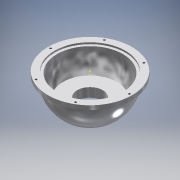
# Autodesk Inventor part: Kugel_unten_V5_leer
Saved by Autodesk Inventor 2016 (Build 200138000, 138)
## iProperties
Created: 2015-06-19
Part Number: Kugel_unten_V5_leer
Material: ABS-Kunststoff
Document SubType Name: Modeling
Designer: Johann
Mass: 41.0322 g
Surface Area: 192.915 cm^2
Volume: 38.7096 cm^3
Density: 1.06 g/cm^3
Appearance: Glatt - weiß
Author: Johann
Autodesk Inventor part; units mm, degrees
ref_plane "YZ Plane" through (0, 0, 0) normal (1, 0, 0) x (0, 1, 0)
sketch "Skizze1" plane through (0, 0, 0) normal (1, 0, 0) x (0, 1, 0)
  line L0 (0, 0) -> (0, 50)
  arc A0 (32.8487, 27.1754) -> (40, 50) centre (0, 50) ccw
  arc A1 (28.5, 15.1754) -> (45, 50) centre (0, 50) ccw
  line L1 (40, 50) -> (40, 55)
  line L2 (40, 55) -> (45, 55)
  line L3 (45, 55) -> (45, 50)
  line L4 (0, 50) -> (40, 50) construction
  line L5 (0, 50) -> (32.8487, 27.1754) construction
  line L6 (28.5, 15.1754) -> (22.5, 15.1754)
  line L7 (22.5, 15.1754) -> (22.5, 17.1754)
  line L8 (22.5, 17.1754) -> (18.5, 17.1754)
  line L9 (18.5, 17.1754) -> (18.5, 15.9754)
  line L10 (18.5, 15.9754) -> (15.5, 15.9754)
  line L11 (15.5, 15.9754) -> (15.5, 27.1754)
  line L12 (15.5, 27.1754) -> (32.8487, 27.1754)
  line L13 (0, 36.0806) -> (37.5, 36.0806) construction
  dimension "d3" = 5
  dimension "r_Kugel" = 45
  dimension "d5" = 50
  dimension "d7" = 5
  dimension "d36" = 4
  dimension "d38" = 2
  dimension "d40" = 1.2
  dimension "d41" = 45
  dimension "d179" = 3
  dimension "d194" = 17.3487
  dimension "d292" = 10
  dimension "d293" = 6
  dimension "d294" = 37.5
  dimension "d295" = 13.9194
  dimension "d296" = 8.9052
  constraints: 28 end point, 6 perpendicular, 6 point on circle, 4 horizontal, 3 coincident, 3 vertical, 2 centre point, 1 point on line, 1 tangent
  measures "d3" radial gap between concentric circles of A1 A0
  measures "r_Kugel" radius of A1
  measures "d5" distance of L0.start L0.end
  measures "d7" distance of L1.start L1.end
  measures "d36" distance of L7.end L8.end
  measures "d38" distance of L6.end L7.end
  measures "d40" distance of L8.end L9.end
  measures "d41" diameter of L7 L0
  measures "d179" distance of L9.end L10.end
  measures "d194" distance of L11.end L5.end
  measures "d292" distance between parallel lines of L12 L8
  measures "d293" distance of L6.start L6.end
  measures "d294" distance of L13.start L13.end
  measures "d295" distance between parallel lines of L4 L13
  measures "d296" distance between parallel lines of L12 L13
revolve "Umdrehung1" add sketch "Skizze1" angle 360 about axis through (0, 0, 0) along (0, 0, 1)
sketch "Skizze6" plane through (0, 0, 27.1754) normal (0, 0, 1) x (1, 0, 0)
  circle A0 centre (0, 0) radius 32.8487 construction
  circle A1 centre (0, 0) radius 15.5 construction
  line L0 (-6.5, -15.5) -> (18.5, -15.5)
  line L1 (18.5, -15.5) -> (18.5, -23.5)
  line L2 (18.5, -23.5) -> (-6.5, -23.5)
  line L3 (-6.5, -23.5) -> (-6.5, -15.5)
  line L4 (-6.5, -23.5) -> (18.5, -15.5) construction
  line L5 (18.5, -23.5) -> (-6.5, -15.5) construction
  circle A2 centre (0, 0) radius 32.8487 projected
  point P0 (0, 0)
  point P1 (6, -15.5)
  point P2 (6, -19.5)
  dimension "d130" = 8
  dimension "d180" = 25
  dimension "d191" = 6
  constraints: 12 end point, 2 midpoint, 2 parallel, 1 horizontal, 1 perpendicular, 1 tangent
  measures "d130" distance of L2.end L0.start
  measures "d180" distance of L0.start L0.end
  measures "d191" horizontal distance of point (0, 0) point (6, -19.5)
ref_plane "Arbeitsebene2" through (0, 0, 31.1754) normal (0, 0, 1) x (1, 0, 0)
sketch "Skizze7" plane through (0, 0, 31.1754) normal (0, 0, 1) x (1, 0, 0)
  line L0 (-6.5, -23.5) -> (-6.5, -15.5) construction
  line L1 (18.5, -23.5) -> (-6.5, -23.5) construction
  line L2 (-6.5, -15.5) -> (18.5, -15.5) construction
  line L3 (18.5, -15.5) -> (18.5, -23.5) construction
  line L4 (18.5, -23.5) -> (-6.5, -15.5) construction
  line L5 (-6.5, -23.5) -> (18.5, -15.5) construction
  line L6 (-0.5, -15.5) -> (19.5, -15.5)
  line L7 (19.5, -15.5) -> (19.5, -20.5)
  line L8 (19.5, -20.5) -> (-0.5, -20.5)
  line L9 (-0.5, -20.5) -> (-0.5, -15.5)
  line L10 (-0.5, -20.5) -> (19.5, -15.5) construction
  line L11 (19.5, -20.5) -> (-0.5, -15.5) construction
  point P0 (0, 0)
  point P1 (6, -19.5)
  point P2 (9.5, -15.5)
  point P3 (9.5, -18)
  dimension "d50" = 20
  dimension "d51" = 5
  dimension "d98" = 25
  dimension "d99" = 8
  dimension "d221" = 1
  constraints: 12 end point, 2 midpoint, 2 parallel, 1 collinear, 1 horizontal, 1 perpendicular
  measures "d50" distance of L7.end L8.end
  measures "d51" distance of L6.end L7.end
  measures "d98" distance of L1.start L0.start
  measures "d99" distance of L2.end L1.start
  measures "d221" distance between parallel lines of L7 L3
ref_plane "Arbeitsebene3" through (0, 0, 41.1754) normal (0, 0, 1) x (1, 0, 0)
sketch "Skizze8" plane through (0, 0, 41.1754) normal (0, 0, 1) x (1, 0, 0)
  point P0 (0, 0)
feature "Erhebung1" [suppressed]
extrude "Extrusion16" [suppressed]
feature "Rippe1" [suppressed]
sketch "Skizze31" plane through (-0.5, -20.5, 41.1754) normal (0, -1, 0) x (1, 0, 0)
  line L0 (0, 0) -> (20, 0) construction
  line L1 (16, 0) -> (4, 0)
  arc A0 (4, 0) -> (16, 0) centre (10, 0) ccw
  point P0 (0.5, -41.1754)
  dimension "d181" = 12
  constraints: 2 end point, 2 midpoint, 2 point on circle, 1 centre point, 1 coincident, 1 horizontal
  measures "d181" distance of L1.start L1.end
extrude "Extrusion17" [suppressed]
sketch "Skizze39" plane through (-0.5, -19.4434, 31.1754) normal (0, 0, 1) x (1, 0, 0)
  arc A0 (-20.4801, -8.9374) -> (-18.1844, -10.4987) centre (0.5, 19.4434) ccw construction
  line L0 (-18.1844, -10.4987) -> (0, 0) construction
  line L1 (0, 2.8868) -> (-20.4801, -8.9374) construction
  arc A1 (8.75, -14.8724) -> (11.25, -14.1732) centre (0.5, 19.4434) ccw construction
  line L2 (11.25, -14.1732) -> (11.25, -1.0566) construction
  line L3 (8.75, -1.0566) -> (8.75, -14.8724) construction
  circle A2 centre (-9.0922, -5.2494) radius 2.5
  circle A3 centre (8.75, -7.9645) radius 2.5
  line L4 (0, 3.9434) -> (20, 3.9434) projected
  line L5 (0, 2.8868) -> (0, 3.9434) projected
  line L6 (0, 2.8868) -> (-20.4801, -8.9374) projected
  arc A4 (-20.4801, -8.9374) -> (-18.1844, -10.4987) centre (0.5, 19.4434) ccw projected
  line L7 (-18.1844, -10.4987) -> (0, 0) projected
  line L8 (0, -1.0566) -> (0, 0) projected
  line L9 (8.75, -1.0566) -> (0, -1.0566) projected
  line L10 (20, -1.0566) -> (11.25, -1.0566) projected
  line L11 (20, 0) -> (20, -1.0566) projected
  line L12 (20, 0) -> (26.8981, -3.9826) projected
  arc A5 (26.8981, -3.9826) -> (28.5115, -2.0274) centre (0.5, 19.4434) ccw projected
  line L13 (28.5115, -2.0274) -> (20, 2.8868) projected
  line L14 (20, 3.9434) -> (20, 2.8868) projected
  line L15 (0, 3.9434) -> (20, 3.9434) projected
  line L16 (0, 2.8868) -> (0, 3.9434) projected
  line L17 (0, -1.0566) -> (0, 0) projected
  line L18 (8.75, -1.0566) -> (0, -1.0566) projected
  line L19 (8.75, -1.0566) -> (8.75, -14.8724) projected
  arc A6 (8.75, -14.8724) -> (11.25, -14.1732) centre (0.5, 19.4434) ccw projected
  line L20 (11.25, -14.1732) -> (11.25, -1.0566) projected
  line L21 (20, -1.0566) -> (11.25, -1.0566) projected
  line L22 (20, 0) -> (20, -1.0566) projected
  line L23 (20, 0) -> (26.8981, -3.9826) projected
  arc A7 (26.8981, -3.9826) -> (28.5115, -2.0274) centre (0.5, 19.4434) ccw projected
  line L24 (28.5115, -2.0274) -> (20, 2.8868) projected
  line L25 (20, 3.9434) -> (20, 2.8868) projected
  dimension "d225" = 5
  constraints: 2 centre point, 2 midpoint, 1 equal radius
  measures "d225" diameter of A2
extrude "Extrusion21" [suppressed]
sketch "Skizze42" plane through (-0.5, -19.4434, 31.1754) normal (0, 0, 1) x (1, 0, 0)
  line L0 (-18.1844, -10.4987) -> (0, 0) construction
  line L1 (0, 2.8868) -> (-20.4801, -8.9374) construction
  arc A0 (-20.4801, -8.9374) -> (-18.1844, -10.4987) centre (0.5, 19.4434) ccw construction
  line L2 (11.25, -14.1732) -> (11.25, -1.0566) construction
  line L3 (8.75, -1.0566) -> (8.75, -14.8724) construction
  arc A1 (8.75, -14.8724) -> (11.25, -14.1732) centre (0.5, 19.4434) ccw construction
  line L4 (0, 3.9434) -> (20, 3.9434) projected
  line L5 (0, 2.8868) -> (0, 3.9434) projected
  line L6 (0, 2.8868) -> (-20.4801, -8.9374) projected
  arc A2 (-20.4801, -8.9374) -> (-18.1844, -10.4987) centre (0.5, 19.4434) ccw projected
  line L7 (-18.1844, -10.4987) -> (0, 0) projected
  line L8 (0, -1.0566) -> (0, 0) projected
  line L9 (8.75, -1.0566) -> (0, -1.0566) projected
  line L10 (20, -1.0566) -> (11.25, -1.0566) projected
  line L11 (20, 0) -> (20, -1.0566) projected
  line L12 (20, 0) -> (26.8981, -3.9826) projected
  arc A3 (26.8981, -3.9826) -> (28.5115, -2.0274) centre (0.5, 19.4434) ccw projected
  line L13 (28.5115, -2.0274) -> (20, 2.8868) projected
  line L14 (20, 3.9434) -> (20, 2.8868) projected
  line L15 (0, 3.9434) -> (20, 3.9434) projected
  line L16 (0, 2.8868) -> (0, 3.9434) projected
  line L17 (0, -1.0566) -> (0, 0) projected
  line L18 (8.75, -1.0566) -> (0, -1.0566) projected
  line L19 (8.75, -1.0566) -> (8.75, -14.8724) projected
  arc A4 (8.75, -14.8724) -> (11.25, -14.1732) centre (0.5, 19.4434) ccw projected
  line L20 (11.25, -14.1732) -> (11.25, -1.0566) projected
  line L21 (20, -1.0566) -> (11.25, -1.0566) projected
  line L22 (20, 0) -> (20, -1.0566) projected
  line L23 (20, 0) -> (26.8981, -3.9826) projected
  arc A5 (26.8981, -3.9826) -> (28.5115, -2.0274) centre (0.5, 19.4434) ccw projected
  line L24 (28.5115, -2.0274) -> (20, 2.8868) projected
  line L25 (20, 3.9434) -> (20, 2.8868) projected
  point P0 (-5.5228, -3.1886)
  point P1 (8.7436, -4.3348)
hole "Bohrung4" [suppressed]
sketch "Skizze32" plane through (0, 0, 41.1754) normal (0, 0, 1) x (1, 0, 0)
  line L0 (3.5, -20.5) -> (3.5, -15.5) construction
  line L1 (3.5, -15.5) -> (-0.5, -15.5) construction
  line L2 (-0.5, -15.5) -> (-0.5, -20.5) construction
  line L3 (-0.5, -20.5) -> (3.5, -20.5) construction
  line L4 (-0.5, -20.5) -> (3.5, -15.5) construction
  line L5 (-0.5, -15.5) -> (3.5, -20.5) construction
  point P0 (0, 0)
  point P1 (1.5, -18)
  constraints: 4 end point, 1 midpoint
hole "Bohrung3" [suppressed]
ref_plane "Arbeitsebene11" through (9.5, -20.5, 41.1754) normal (1, 0, 0) x (0, 0, -1)
mirror "Spiegeln6" [suppressed]
mirror "Spiegeln3" [suppressed]
sketch "Skizze36" plane through (-6.5, -15.5, 27.1754) normal (0, 0, 1) x (1, 0, 0)
  circle A0 centre (6.5, 15.5) radius 15.5 construction
  circle A1 centre (6.5, 15.5) radius 32.8487 construction
  circle A2 centre (-7.1511, -1.4325) radius 5.25
  line L0 (-7.1511, -1.4325) -> (-7.8178, 4.7818) construction
  line L1 (-7.8178, 4.7818) -> (-7.7112, 3.7875)
  arc A3 (-13.3654, -2.0993) -> (-7.8178, 4.7818) centre (-7.1511, -1.4325) ccw
  line L2 (-7.1511, -1.4325) -> (-13.3654, -2.0993) construction
  line L3 (-13.3654, -2.0993) -> (-12.3711, -1.9926)
  arc A4 (6.5, 31) -> (6.5, 0) centre (6.5, 15.5) ccw projected
  arc A5 (1.5102, 36.6699) -> (1.5102, -5.6699) centre (6.5, 15.5) ccw construction
  arc A6 (-18.6964, 10.2798) -> (-16.1571, 3.3029) centre (-13.9383, 8.0611) ccw
  line L4 (-13.9383, 8.0611) -> (-18.6964, 10.2798) construction
  line L5 (-13.9383, 8.0611) -> (-16.1571, 3.3029) construction
  arc A7 (-9.1802, 5.8423) -> (-11.7196, 12.8192) centre (-13.9383, 8.0611) ccw
  line L6 (-13.9383, 8.0611) -> (-11.7196, 12.8192) construction
  line L7 (-13.9383, 8.0611) -> (-9.1802, 5.8423) construction
  arc A8 (-16.1571, 3.3029) -> (-9.1802, 5.8423) centre (-13.9383, 8.0611) ccw
  arc A9 (-11.7196, 12.8192) -> (-18.6964, 10.2798) centre (-13.9383, 8.0611) ccw
  line L8 (6.5, 15.5) -> (-15.25, 15.5) construction
  arc A10 (-8.2739, 5.4197) -> (-11.297, 13.7255) centre (-13.9383, 8.0611) ccw
  line L9 (-9.1802, 5.8423) -> (-8.2739, 5.4197)
  line L10 (-11.297, 13.7255) -> (-11.7196, 12.8192)
  arc A11 (-19.6027, 10.7024) -> (-16.5797, 2.3966) centre (-13.9383, 8.0611) ccw
  line L11 (-16.1571, 3.3029) -> (-16.5797, 2.3966)
  line L12 (-18.6964, 10.2798) -> (-19.6027, 10.7024)
  circle A12 centre (-7.1511, 32.4325) radius 5.25
  line L13 (-7.1511, 32.4325) -> (-7.8178, 26.2182) construction
  line L14 (-7.1511, 32.4325) -> (-13.3654, 33.0993) construction
  line L15 (-7.1511, 32.4325) -> (-7.8178, 26.2182) construction
  arc A13 (-16.1571, 27.6971) -> (-18.6964, 20.7202) centre (-13.9383, 22.9389) ccw
  line L16 (-13.9383, 22.9389) -> (-18.6964, 20.7202) construction
  line L17 (-13.9383, 22.9389) -> (-16.1571, 27.6971) construction
  arc A14 (-11.7196, 18.1808) -> (-9.1802, 25.1577) centre (-13.9383, 22.9389) ccw
  line L18 (-13.9383, 22.9389) -> (-11.7196, 18.1808) construction
  line L19 (-13.9383, 22.9389) -> (-9.1802, 25.1577) construction
  arc A15 (-9.1802, 25.1577) -> (-16.1571, 27.6971) centre (-13.9383, 22.9389) ccw
  arc A16 (-18.6964, 20.7202) -> (-11.7196, 18.1808) centre (-13.9383, 22.9389) ccw
  line L20 (-12.1427, 27.8723) -> (-15.7339, 18.0056) construction
  arc A17 (-11.297, 17.2745) -> (-8.2739, 25.5803) centre (-13.9383, 22.9389) ccw
  line L21 (-9.1802, 25.1577) -> (-8.2739, 25.5803)
  line L22 (-11.297, 17.2745) -> (-11.7196, 18.1808)
  arc A18 (-16.5797, 28.6034) -> (-19.6027, 20.2976) centre (-13.9383, 22.9389) ccw
  line L23 (-16.1571, 27.6971) -> (-16.5797, 28.6034)
  line L24 (-18.6964, 20.7202) -> (-19.6027, 20.2976)
  line L25 (-12.1427, 3.1277) -> (-15.7339, 12.9944) construction
  line L26 (-11.2382, 1.8626) -> (-3.0639, -4.7276) construction
  line L27 (-11.2382, 29.1374) -> (-3.0639, 35.7276) construction
  arc A19 (-7.8178, 26.2182) -> (-13.3654, 33.0993) centre (-7.1511, 32.4325) ccw
  line L28 (-7.8178, 26.2182) -> (-7.7112, 27.2125)
  line L29 (-12.3711, 32.9926) -> (-13.3654, 33.0993)
  dimension "Durchmesser_Bat" = 10.5
  dimension "d203" = 90
  dimension "d206" = 90
  dimension "d207" = 5.25
  dimension "d208" = 90
  dimension "d209" = 20
  dimension "d210" = 90
  dimension "d266" = 1
  constraints: 60 end point, 45 point on circle, 22 symmetric about line, 17 centre point, 16 coincident, 5 tangent, 4 collinear, 4 midpoint, 4 point on line, 2 concentric, 2 equal length, 1 horizontal, 1 horizontal alignment, 1 vertical alignment, 9 other
  measures "Durchmesser_Bat" diameter of A2
  measures "d203" angle of L0 L2
  measures "d206" angle of L4 L5
  measures "d207" radius of A7
  measures "d208" angle of L7 L6
  measures "d210" angle of L6 L4
  measures "d266" radial gap between concentric circles of A2 A3
extrude "Extrusion18" [suppressed]
extrude "Extrusion20" [suppressed]
sketch "Skizze37" plane through (0, -15.5, 27.1754) normal (0, 0, 1) x (1, 0, 0)
  circle A0 centre (0, 15.5) radius 15.5 construction
  circle A1 centre (0, 15.5) radius 32.8487 construction
  circle A2 centre (19.1833, 5.25) radius 5.25
  arc A3 (15.8821, 10.557) -> (25.4299, 5.4554) centre (19.1833, 5.25) ccw
  line L0 (19.1833, 5.25) -> (15.8821, 10.557) construction
  line L1 (19.1833, 5.25) -> (25.4299, 5.4554) construction
  line L2 (15.8821, 10.557) -> (16.4103, 9.7079)
  line L3 (25.4299, 5.4554) -> (24.4305, 5.4226)
  arc A4 (15.2582, 0) -> (15.2582, 31) centre (0, 15.5) ccw construction
  line L4 (16.7092, 0.6195) -> (21.6575, 9.8805) construction
  line L5 (0, 15.5) -> (32.8487, 15.5) construction
  arc A5 (0, 48.3487) -> (0, 48.3487) centre (0, 15.5) ccw construction
  circle A6 centre (19.1833, 25.75) radius 5.25
  arc A7 (25.4299, 25.5446) -> (15.8821, 20.443) centre (19.1833, 25.75) ccw
  line L6 (15.8821, 20.443) -> (16.4103, 21.2921)
  line L7 (25.4299, 25.5446) -> (24.4305, 25.5774)
  circle A8 centre (21.75, 15.5) radius 5.25
  arc A9 (17.3306, 19.9194) -> (17.3306, 11.0806) centre (21.75, 15.5) ccw
  arc A10 (26.1694, 11.0806) -> (26.1694, 19.9194) centre (21.75, 15.5) ccw
  line L8 (17.3306, 11.0806) -> (26.1694, 19.9194) construction
  line L9 (26.1694, 11.0806) -> (17.3306, 19.9194) construction
  line L10 (18.0377, 11.7877) -> (17.3306, 11.0806)
  line L11 (18.0377, 19.2123) -> (17.3306, 19.9194)
  line L12 (26.1694, 19.9194) -> (25.4623, 19.2123)
  line L13 (26.1694, 11.0806) -> (25.4623, 11.7877)
  line L14 (21.75, 10.25) -> (21.75, 20.75) construction
  point P0 (20.6457, -1.166)
  point P1 (18.5, -3.5197)
  dimension "d211" = 10.5
  dimension "d214" = 1
  dimension "d218" = 120
  dimension "d220" = 90
  constraints: 30 end point, 27 point on circle, 8 centre point, 7 collinear, 6 symmetric about line, 5 coincident, 4 midpoint, 3 tangent, 2 equal radius, 2 point on line, 1 equal length, 1 horizontal, 1 vertical, 6 other
  measures "d211" diameter of A2
  measures "d214" radial gap between concentric circles of A3 A2
  measures "d218" angle of L1 L0
  measures "d220" angle of L8 L9
extrude "Extrusion19" [suppressed]
extrude "Extrusion22" [suppressed]
ref_plane "Arbeitsebene13" through (0, 0, 32.1754) normal (0, 0, 1) x (0, -1, 0)
sketch "Skizze44" plane through (0, 0, 32.1754) normal (0, 0, 1) x (0, -1, 0)
  circle A0 centre (0, 0) radius 15.5 construction
  circle A1 centre (0, 0) radius 15.5 construction
  line L0 (-0.8, -2) -> (-3.8, -2)
  line L1 (-3.8, -2) -> (-3.8, 2)
  line L2 (-3.8, 2) -> (-0.8, 2)
  line L3 (-0.8, 4) -> (-5.8, 4)
  line L4 (-5.8, 4) -> (-5.8, -4)
  line L5 (-5.8, -4) -> (-0.8, -4)
  line L6 (-0.8, -2) -> (-0.8, -4)
  line L7 (-0.8, 2) -> (-0.8, 4)
  point P0 (0, 0)
  point P1 (-3.8, 0)
  dimension "d245" = 2
  dimension "d246" = 4
  dimension "d247" = 3
  dimension "d277" = 0.8
  constraints: 16 end point, 4 perpendicular, 2 vertical, 1 collinear, 1 horizontal, 1 horizontal alignment, 1 midpoint, 2 other
  measures "d245" distance between parallel lines of L1 L4
  measures "d246" distance of L0.end L1.end
  measures "d247" distance of L0.start L0.end
  measures "d277" distance from line of L7 point (0, 0)
extrude "Extrusion23" [suppressed]
sketch "Skizze46" plane through (-5.8, 4, 41.1754) normal (0, 0, 1) x (1, 0, 0)
  line L0 (0, -8) -> (5, -8)
  line L1 (1, -8) -> (4, -8)
  line L2 (4, -8) -> (8.3, -19.5)
  line L3 (1, -8) -> (5.3, -19.5)
  line L4 (5.3, -19.5) -> (8.3, -19.5)
  line L5 (5, -6) -> (5, -8) construction
  line L6 (2, -6) -> (5, -6) construction
  line L7 (2, -2) -> (2, -6) construction
  line L8 (5, -2) -> (2, -2) construction
  line L9 (5, 0) -> (5, -2) construction
  line L10 (0, 0) -> (5, 0) construction
  line L11 (0, -8) -> (0, 0) construction
  line L12 (5, -8) -> (0, -8) construction
  line L13 (5.8, -19.5) -> (24.3, -19.5) construction
  line L14 (-0.7, -19.5) -> (5.8, -19.5) construction
  line L15 (-0.7, -19.5) -> (5.3, -19.5) construction
  line L16 (5.3, -19.5) -> (5.3, -24.5) construction
  line L17 (0, -8) -> (0, 0) construction
  line L18 (5, -8) -> (0, -8) construction
  circle A0 centre (5.8, -4) radius 40 construction
  circle A1 centre (5.8, -4) radius 32.8487 construction
  line L19 (0, -5.5) -> (-34.2, -5.5)
  line L20 (-34.2, -5.5) -> (-34.2, -4)
  line L21 (-34.2, -4) -> (0, -4)
  line L22 (0, -4) -> (0, -5.5)
  line L23 (24.3, -19.5) -> (25.3, -19.5) projected
  line L24 (5.3, -19.5) -> (25.3, -19.5) projected
  point P0 (2, -4)
  point P1 (-17.1, -4)
  dimension "d252" = 3
  dimension "d253" = 1
  dimension "d255" = 5
  dimension "d268" = 1.5
  constraints: 18 end point, 3 parallel, 3 point on line, 2 collinear, 2 horizontal, 2 midpoint, 1 horizontal alignment, 1 perpendicular, 1 tangent
  measures "d252" distance of L1.start L1.end
  measures "d253" distance of L0.start L1.start
  measures "d255" distance of L0.end L0.start
  measures "d268" distance between parallel lines of L21 L19
extrude "Extrusion24" [suppressed]
chamfer "Fase3" [suppressed]
chamfer "Fase2" [suppressed]
mirror "Spiegeln8" [suppressed]
ref_plane "Arbeitsebene14" through (19.5, -15.5, 41.1754) normal (0, 1, 0) x (1, 0, 0)
ref_plane "Arbeitsebene1" through (0, 45, 50) normal (0, 1, 0) x (-1, 0, 0)
sketch "Skizze13" plane through (0, 0, 15.1754) normal (0, 0, -1) x (-1, 0, 0)
  circle A0 centre (0, 0) radius 22.5 construction
  circle A1 centre (0, 0) radius 25.5 construction
  point P0 (0, 0)
  point P1 (-25.5, 0)
  point P2 (-12.75, -22.0836)
  point P3 (12.75, -22.0836)
  point P4 (25.5, 0)
  point P5 (12.75, 22.0836)
  point P6 (-12.75, 22.0836)
  dimension "d82" = 51
  dimension "d83" = 45
  dimension "d87" = 360
  constraints: 2 horizontal alignment, 1 coincident, 9 other
  measures "d83" diameter of A0
hole "Bohrung1" at (25.5, 0, 15.1754) at (12.75, -22.0836, 15.1754) at (-12.75, -22.0836, 15.1754) at (-25.5, 0, 15.1754) at (-12.75, 22.0836, 15.1754) at (12.75, 22.0836, 15.1754) direction (0, 0, 1) diameter 2.459 depth 10 tip angle 118 thread size "M3x0.5" class "6H" standard "ISO Metric profile"
ref_plane "Arbeitsebene17" through (15.5, -15.5, 41.1754) normal (0, 1, 0) x (1, 0, 0)
sketch "Skizze53" plane through (15.5, -15.5, 41.1754) normal (0, 1, 0) x (1, 0, 0)
  arc A0 (0, 0) -> (-12, 0) centre (-6, 0) ccw construction
  circle A1 centre (-6, 0) radius 8.5
  point P0 (-15.5, 41.1754)
  dimension "d304" = 17
  constraints: 1 centre point, 1 coincident
  measures "d304" diameter of A1
extrude "Extrusion29" [suppressed]
sketch "Skizze52" plane through (0, 0, 27.1754) normal (0, 0, 1) x (0, -1, 0)
  circle A0 centre (0, 0) radius 32.8487 construction
  circle A1 centre (0, 0) radius 15.5 projected
  line L0 (15.5, 0) -> (12.7669, 15.5)
  line L1 (15.5, 0) -> (12.7669, -15.5)
  line L2 (3.8874, -15.5) -> (15.5, -15.5) projected
  line L3 (15.5, 0) -> (0, 0) construction
  line L4 (12.7669, 15.5) -> (-15.5, 15.5)
  line L5 (-15.5, 15.5) -> (-15.5, 18.9793)
  line L6 (-5.701, 2.0068) -> (19.5, 16.5566) projected
  line L7 (12.7669, -15.5) -> (12.7669, 18.0207)
  line L8 (12.7669, 18.0207) -> (15.5, 18.0207)
  line L9 (19.5, -16.5566) -> (1.5276, -6.1802) projected
  arc A2 (29.5385, -23.1026) -> (29.5385, 23.1026) centre (0, 0) ccw
  line L10 (0, 0) -> (29.5385, 23.1026) construction
  line L11 (0, 0) -> (29.5385, -23.1026) construction
  line L12 (-15.5, 18.9793) -> (29.5385, 23.1026)
  line L13 (15.5, 18.0207) -> (29.5385, -23.1026)
  arc A3 (14.5652, -5.3013) -> (14.5652, 5.3013) centre (0, 0) ccw
  circle A4 centre (0, 0) radius 15.5 projected
  point P0 (0, 0)
  point P1 (2.883, 15.2295)
  point P2 (2.883, -15.2295)
  point P3 (-20.3813, 15.9406)
  point P4 (-20.3813, -15.9406)
  point P5 (3.5, -15.5)
  dimension "d297" = 160
  dimension "d298" = 37.5
  constraints: 22 end point, 6 point on circle, 5 point on line, 2 centre point, 2 coincident, 2 horizontal, 2 perpendicular, 1 equal length, 1 other
  measures "d297" angle of L1 L0
  measures "d298" radius of A2
extrude "Extrusion28" [suppressed]
sketch "Skizze54" plane through (0, 0, 0) normal (0, 1, 0) x (-1, 0, 0)
  arc A0 (-15.5, 41.1754) -> (-3.5, 41.1754) centre (-9.5, 41.1754) ccw construction
  circle A1 centre (-9.5, 41.1754) radius 11
  line L0 (-9.5, 52.1754) -> (-9.5, 30.1754)
  point P0 (0, 0)
  point P1 (-3.8874, 39.0544)
  dimension "d310" = 22
  constraints: 2 coincident, 2 end point, 2 point on circle, 1 centre point, 1 midpoint, 1 vertical
  measures "d310" diameter of A1
extrude "Extrusion31" [suppressed]
ref_plane "Arbeitsebene18" through (9.5, -15.5, 41.1754) normal (0, 1, 0) x (1, 0, 0)
sketch "Skizze55" plane through (0, -2.5, 0) normal (0, 1, 0) x (1, 0, 0)
  arc A0 (19.249, -36.0806) -> (15.2971, -31.827) centre (9.5, -41.1754) ccw construction
  circle A1 centre (9.5, -41.1754) radius 11
  line L0 (9.5, -30.1754) -> (9.5, -52.1754)
  point P0 (0, 0)
  constraints: 2 end point, 2 point on circle, 1 centre point, 1 coincident, 1 concentric, 1 midpoint, 1 vertical
feature "Erhebung3" [suppressed]
ref_plane "Arbeitsebene19" through (0, 0, 36.0806) normal (0, 0, 1) x (1, 0, 0)
sketch "Skizze57" plane through (0, 0, 36.0806) normal (0, 0, 1) x (1, 0, 0)
  circle A0 centre (20.1266, 10.0318) radius 5.25 construction
  line L0 (19.5, -15.5) -> (16.3039, -15.5) construction
  line L1 (19.5, -16.6246) -> (19.5, -15.5) construction
  line L2 (19.5, -16.6246) -> (29.5385, -23.1026) construction
  arc A1 (29.5385, -23.1026) -> (29.5385, 23.1026) centre (0, 0) ccw construction
  line L3 (29.5385, 23.1026) -> (19.5, 16.6246) construction
  line L4 (19.5, 15.5) -> (19.5, 16.6246) construction
  line L5 (12.7669, 15.5) -> (19.5, 15.5) construction
  line L6 (12.7669, 15.5) -> (14.5652, 5.3013) construction
  arc A2 (15.2971, 2.5) -> (14.5652, 5.3013) centre (0, 0) ccw construction
  line L7 (15.2971, 2.5) -> (19.249, 2.5) construction
  line L8 (19.249, 2.5) -> (19.249, -2.5) construction
  circle A3 centre (32.028, -4.0447) radius 5.25 construction
  circle A4 centre (23.1718, -11.3161) radius 5.25 construction
  circle A5 centre (31.4376, 7.173) radius 5.25 construction
  point P0 (0, 0)
  dimension "d318" = 10.5
  constraints: 4 centre point, 3 equal radius, 1 other
  measures "d318" diameter of A0
ref_plane "Arbeitsebene16" through (0, 0, 55) normal (0, 0, 1) x (1, 0, 0)
sketch "Skizze60" plane through (0, 0, 55) normal (0, 0, 1) x (1, 0, 0)
  circle A0 centre (0, 0) radius 45 construction
  circle A1 centre (49, 0) radius 4
  spline S0 degree 4 poles (53, 0) (53, 3.9822) (49.4674, 8.0628) (44.676, 6.3897) (43.9333, 9.7398) knots 0 0 0 0 0 1 1 1 1 1
  arc A2 (43.9333, -9.7398) -> (43.9333, 9.7398) centre (0, 0) ccw
  line L0 (43.9333, 9.7398) -> (0, 0) construction
  line L1 (0, 0) -> (43.9333, -9.7398) construction
  line L2 (0, 0) -> (45, 0) construction
  spline S1 degree 4 poles (43.9333, -9.7398) (44.676, -6.3897) (49.4674, -8.0628) (53, -3.9822) (53, 0) knots 0 0 0 0 0 1 1 1 1 1
  point P0 (48.4333, 6.5398)
  point P1 (48.4333, -6.5398)
  dimension "d326" = 8
  dimension "d327" = 25
  dimension "d328" = 3.2
  dimension "d329" = 4.5
  dimension "d330" = 4.5
  dimension "d331" = 3.2
  constraints: 6 end point, 5 point on circle, 3 horizontal alignment, 1 centre point, 1 coincident, 1 concentric, 1 horizontal, 12 other
  measures "d327" angle of L1 L0
  measures "d328" vertical distance of L0.start point (48.433, 6.54)
  measures "d329" horizontal distance of L0.start point (48.433, 6.54)
  measures "d330" horizontal distance of L1.end point (48.433, -6.54)
  measures "d331" vertical distance of L1.end point (48.433, -6.54)
extrude "Extrusion32" [suppressed]
sketch "Skizze61" plane through (0, 0, 50) normal (0, 0, -1) x (-1, 0, 0)
  spline S0 degree 4 poles (-43.9333, 9.7398) (-44.676, 6.3897) (-49.4674, 8.0628) (-53, 3.9822) (-53, 0) knots -1 -1 -1 -1 -1 0 0 0 0 0
  spline S1 degree 4 poles (-53, 0) (-53, -3.9822) (-49.4673, -8.0628) (-44.676, -6.3897) (-43.9333, -9.7398) knots -1 -1 -1 -1 -1 0 0 0 0 0
  arc A0 (-43.9333, 9.7398) -> (-43.9333, -9.7398) centre (0, 0) ccw construction
  circle A1 centre (-49, 0) radius 4 construction
  arc A2 (-43.9333, 9.7398) -> (-43.9333, -9.7398) centre (0, 0) ccw construction
  line L0 (-52.3775, -2.75) -> (-47.8377, -2.75)
  line L1 (-47.8377, -2.75) -> (-46.25, 0)
  line L2 (-46.25, 0) -> (-47.8377, 2.75)
  line L3 (-47.8377, 2.75) -> (-52.3775, 2.75)
  line L4 (-49, 0) -> (-53, 0) construction
  dimension "d334" = 5.5
  dimension "d335" = 120
  dimension "d336" = 2.3816
  constraints: 10 end point, 4 point on circle, 2 centre point, 2 equal length, 2 horizontal, 1 horizontal alignment, 1 parallel, 12 other
  measures "d334" distance between parallel lines of L3 L0
  measures "d335" angle of L0 L1
  measures "d336" distance from line of L4.start L1
extrude "Extrusion34" [suppressed]
hole "Bohrung5" [suppressed]
pattern_circular "Runde Anordnung1" [suppressed]
sketch "Skizze62" plane through (0, 0, 55) normal (0, 0, 1) x (1, 0, 0)
  point P0 (0, 0)
sketch "Skizze63" plane through (0, 0, 55) normal (0, 0, 1) x (1, 0, 0)
  circle A0 centre (0, 0) radius 45 projected
  circle A1 centre (0, 0) radius 40 projected
  circle A2 centre (0, 0) radius 51
  dimension "d351" = 102
  constraints: 1 centre point, 1 coincident
  measures "d351" diameter of A2
extrude "Extrusion35" add sketch "Skizze63" against normal blind 5 contours A2
sketch "Skizze64" plane through (0, 0, 55) normal (0, 0, 1) x (1, 0, 0)
  circle A0 centre (0, 0) radius 51 projected
  circle A1 centre (0, 0) radius 40 projected
  circle A2 centre (0, 0) radius 43
  dimension "d354" = 86
  constraints: 1 centre point, 1 coincident
  measures "d354" diameter of A2
extrude "Extrusion36" cut sketch "Skizze64" against normal blind 2 contours A2
sketch "Skizze65" plane through (0, 0, 55) normal (0, 0, 1) x (1, 0, 0)
  point P0 (0, 0)
  point P1 (-48, 0)
  dimension "d357" = 48
  measures "d357" distance of point (-48, 0) point (0, 0)
hole "Bohrung6" at (-48, 0, 55) direction (0, 0, -1) diameter 2.459 end through all thread size "M3x0.5" class "6H" standard "ISO Metric profile"
pattern_circular "Runde Anordnung2" count 6 over 360 about axis through (0, 0, 55) along (0, 0, -1) of "Bohrung6"
ref_plane "Arbeitsebene20" through (0, 0, 30) normal (0, 0, -1) x (-1, 0, 0)
sketch "Skizze9" plane through (0, 0, 31.1754) normal (0, 0, 1) x (1, 0, 0)
  circle A0 centre (0, 0) radius 40 construction
  circle A1 centre (0, 0) radius 32.8487 construction
  line L0 (18.5, -23.5) -> (-6.5, -23.5) construction
  line L1 (-6.5, -23.5) -> (-0.5, -20.5) construction
  line L2 (9.5, -20.5) -> (9.5, -38.8555)
  line L3 (-6.5, -23.5) -> (-6.5, -15.5) construction
  line L4 (-6.5, -23.5) -> (-0.5, -20.5) construction
  line L5 (-6.5, -15.5) -> (-0.5, -15.5) construction
  line L6 (-0.5, -18) -> (-24.3237, -31.7546)
  line L7 (18.5, -15.5) -> (18.5, -23.5) construction
  line L8 (18.5, -15.5) -> (19.5, -15.5) projected
  line L9 (19.5, -18) -> (31.3508, -24.8421)
  line L10 (18.5, -23.5) -> (19.5, -20.5) projected
  line L11 (18.5, -23.5) -> (19.5, -20.5) projected
  line L12 (-0.5, -20.5) -> (-0.5, -15.5) projected
  line L13 (19.5, -20.5) -> (-0.5, -20.5) projected
  line L14 (19.5, -15.5) -> (19.5, -20.5) projected
  dimension "d62" = 60
  dimension "d224" = 60
  constraints: 6 end point, 3 point on circle, 1 vertical
  measures "d62" angle of L2 L6
  measures "d224" angle of L9 L2
sketch "Skizze56" plane through (9.5, -15.5, 41.1754) normal (0, 1, 0) x (1, 0, 0)
  line L0 (-9.5, 14) -> (9, 14) construction
  circle A0 centre (0, 0) radius 8.5
  line L1 (-3.0048, 7.9512) -> (-3.0048, -7.9512)
  line L2 (30.5, -8.8246) -> (-49.5, -8.8246) projected
  line L3 (-16, 14) -> (-10, 10) projected
  line L4 (9, 14) -> (10, 10) projected
  line L5 (-16, 14) -> (-9.5, 14) projected
  line L6 (-10, 10) -> (10, 10) projected
  point P0 (-9.5, 41.1754)
  point P1 (-3.0048, -0.2722)
  dimension "d313" = 17
  constraints: 2 end point, 2 point on circle, 1 centre point, 1 perpendicular, 1 point on line
  measures "d313" diameter of A0
